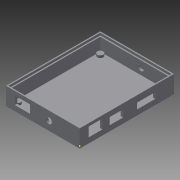
# Autodesk Inventor part: pcbProtectiveCase
Saved by Autodesk Inventor 2015 (Build 190159000, 159)
## iProperties
Created: 2015-02-12
Part Number: pcbProtectiveCase
Material: Generic
Document SubType Name: Modeling
Designer: 477grp12
Density: 1 g/cm^3
Appearance: Default
Author: 477grp12
Autodesk Inventor part; units mm, degrees
ref_plane "YZ Plane" through (0, 0, 0) normal (1, 0, 0) x (0, 1, 0)
ref_plane "XZ Plane" through (0, 0, 0) normal (0, 1, 0) x (-1, 0, 0)
ref_plane "XY Plane" through (0, 0, 0) normal (0, 0, 1) x (1, 0, 0)
sketch "Sketch1" plane through (0, 0, 0) normal (0, 1, 0) x (-1, 0, 0)
  line L0 (0, 0) -> (62.86, 0)
  line L1 (62.86, 0) -> (62.86, -80.39)
  line L2 (62.86, -80.39) -> (0, -80.39)
  line L3 (0, -80.39) -> (0, 0)
  line L4 (2, -2) -> (60.86, -2)
  line L5 (60.86, -2) -> (60.86, -78.39)
  line L6 (60.86, -78.39) -> (2, -78.39)
  line L7 (2, -78.39) -> (2, -2)
  dimension "d0" = 62.86
  dimension "d1" = 80.39
  dimension "d2" = 58.86
  dimension "d3" = 76.39
  dimension "d4" = 2
  dimension "d5" = 2
  constraints: 16 end point, 4 parallel, 2 horizontal, 2 perpendicular
  measures "d0" distance of L1.end L2.end
  measures "d1" distance of L2.end L0.start
  measures "d2" distance of L5.end L6.end
  measures "d3" distance of L4.end L5.end
  measures "d4" distance between parallel lines of L0 L4
  measures "d5" distance between parallel lines of L7 L3
extrude "Extrusion1" add sketch "Sketch1" along normal blind 15 contours L0 L1 L2 L3 | L4 L5 L6 L7
shell "Shell1" thickness 2 removed faces 1 at (-20.9533, 15, -26.7967)
sketch "Sketch2" plane through (-60.86, 2, -2) normal (0, 1, 0) x (1, 0, 0)
  point P0 (60.86, -2)
sketch "Sketch3" plane through (0, 15, 0) normal (0, 1, 0) x (1, 0, 0)
  line L0 (-60.86, 2) -> (-60.86, 78.39) projected
  line L1 (-60.86, 78.39) -> (-2, 78.39) projected
  line L2 (-2, 78.39) -> (-2, 2) projected
  line L3 (-2, 2) -> (-60.86, 2) projected
  line L4 (-62.86, 0) -> (0, 0) projected
  line L5 (0, 0) -> (0, 80.39) projected
  line L6 (0, 80.39) -> (-62.86, 80.39) projected
  line L7 (-62.86, 80.39) -> (-62.86, 0) projected
  line L8 (-61.86, 79.39) -> (-1, 79.39)
  line L9 (-1, 79.39) -> (-1, 1)
  line L10 (-1, 1) -> (-61.86, 1)
  line L11 (-61.86, 1) -> (-61.86, 79.39)
  dimension "d9" = 1
  dimension "d10" = 1
  dimension "d11" = 1
  dimension "d12" = 1
  constraints: 8 end point, 2 parallel, 1 horizontal, 1 perpendicular
  measures "d9" distance between parallel lines of L6 L8
  measures "d10" distance between parallel lines of L5 L9
  measures "d11" distance between parallel lines of L4 L10
  measures "d12" distance between parallel lines of L7 L11
extrude "Extrusion2" cut sketch "Sketch3" against normal blind 2 contours L8 L9 L10 L11
sketch "Sketch4" plane through (-60.86, 2, -2) normal (0, 1, 0) x (1, 0, 0)
  circle A0 centre (3, 73.39) radius 2.5
  circle A1 centre (55.86, 73.39) radius 2.5
  circle A2 centre (3, 3) radius 2.5
  circle A3 centre (55.86, 3) radius 2.5
  line L0 (60.86, 78.39) -> (-2, 78.39) projected
  line L1 (-2, 78.39) -> (-2, -2) projected
  line L2 (60.86, -2) -> (60.86, 78.39) projected
  line L3 (-2, -2) -> (60.86, -2) projected
  dimension "d15" = 5
  dimension "d16" = 5
  dimension "d17" = 5
  dimension "d18" = 5
  dimension "d19" = 5
  dimension "d20" = 5
  dimension "d21" = 5
  dimension "d22" = 5
  dimension "d23" = 5
  dimension "d24" = 5
  dimension "d25" = 5
  dimension "d26" = 5
  constraints: 4 centre point
  measures "d15" distance from line of L0 A0.centre
  measures "d16" distance from line of L1 A0.centre
  measures "d17" distance from line of L2 A1.centre
  measures "d18" distance from line of L0 A1.centre
  measures "d19" distance from line of L3 A3.centre
  measures "d20" distance from line of L2 A3.centre
  measures "d21" distance from line of L1 A2.centre
  measures "d22" distance from line of L3 A2.centre
  measures "d23" diameter of A0
  measures "d24" diameter of A2
  measures "d25" diameter of A3
  measures "d26" diameter of A1
extrude "Extrusion3" add sketch "Sketch4" along normal blind 2 contours A0 | A1 | A2 | A3
sketch "Sketch5" plane through (0, 0, 0) normal (1, 0, 0) x (0, 0, -1)
  line L0 (7.5, 4) -> (2.5, 4) projected
  line L1 (77.89, 4) -> (72.89, 4) projected
  line L2 (72.89, 2) -> (72.89, 4) projected
  line L3 (77.89, 2) -> (77.89, 4) projected
  line L4 (78.39, 2) -> (2, 2) projected
  line L5 (78.39, 2) -> (78.39, 13) projected
  line L6 (80.39, 0) -> (0, 0) projected
  line L7 (80.39, 0) -> (80.39, 15) projected
  line L8 (0, 15) -> (80.39, 15) projected
  line L9 (0, 0) -> (0, 15) projected
  line L10 (7.5, 2) -> (7.5, 4) projected
  line L11 (2, 2) -> (2, 13) projected
  line L12 (2.5, 2) -> (2.5, 4) projected
  line L13 (79.39, 13) -> (1, 13) projected
  line L14 (7.5, 12.508) -> (19.3903, 12.508)
  line L15 (19.3903, 12.508) -> (19.3903, 4.508)
  line L16 (19.3903, 4.508) -> (7.5, 4.508)
  line L17 (7.5, 4.508) -> (7.5, 12.508)
  line L18 (25.6078, 10.508) -> (36.9891, 10.508)
  line L19 (36.9891, 10.508) -> (36.9891, 4.508)
  line L20 (36.9891, 4.508) -> (25.6078, 4.508)
  line L21 (25.6078, 4.508) -> (25.6078, 10.508)
  line L22 (49.0027, 9.508) -> (64.4938, 9.508)
  line L23 (64.4938, 9.508) -> (64.4938, 4.508)
  line L24 (64.4938, 4.508) -> (49.0027, 4.508)
  line L25 (49.0027, 4.508) -> (49.0027, 9.508)
  dimension "d29" = 0.508
  dimension "d30" = 8
  dimension "d31" = 6
  dimension "d32" = 5
  constraints: 24 end point, 6 parallel, 3 horizontal, 3 perpendicular, 1 collinear, 1 point on line
  measures "d29" distance between parallel lines of L0 L16
  measures "d30" distance between parallel lines of L16 L14
  measures "d31" distance between parallel lines of L20 L18
  measures "d32" distance between parallel lines of L24 L22
extrude "Extrusion4" cut sketch "Sketch5" against normal blind 2 contours L14 L15 L16 L17 | L18 L19 L20 L21 | L22 L23 L24 L25
sketch "Sketch6" plane through (-62.86, 0, 0) normal (0, 0, 1) x (1, 0, 0)
  line L0 (60.86, 2) -> (2, 2) projected
  line L1 (7.5, 4) -> (2.5, 4) projected
  line L2 (7.5, 2) -> (7.5, 4) projected
  line L3 (2.5, 2) -> (2.5, 4) projected
  line L4 (60.86, 2) -> (60.86, 13) projected
  line L5 (60.36, 4) -> (55.36, 4) projected
  line L6 (55.36, 2) -> (55.36, 4) projected
  line L7 (60.36, 2) -> (60.36, 4) projected
  line L8 (2, 2) -> (2, 13) projected
  line L9 (61.86, 13) -> (1, 13) projected
  line L10 (7.5, 11.508) -> (20.3381, 11.508)
  line L11 (20.3381, 11.508) -> (20.3381, 4.508)
  line L12 (20.3381, 4.508) -> (7.5, 4.508)
  line L13 (7.5, 4.508) -> (7.5, 11.508)
  circle A0 centre (36.6004, 7.508) radius 2.5
  point P0 (62.86, 0)
  dimension "d35" = 0.508
  dimension "d36" = 7
  dimension "d37" = 5
  dimension "d38" = 5.508
  constraints: 8 end point, 2 parallel, 1 centre point, 1 horizontal, 1 perpendicular
  measures "d35" distance between parallel lines of L1 L12
  measures "d36" distance between parallel lines of L12 L10
  measures "d37" diameter of A0
  measures "d38" distance from line of L0 A0.centre
extrude "Extrusion5" cut sketch "Sketch6" against normal blind 2 contours L10 L11 L12 L13 | A0
sketch "Sketch7" plane through (0, 0, -80.39) normal (0, 0, -1) x (-1, 0, 0)
  circle A0 centre (26.2596, 7.508) radius 2.5 projected
  point P0 (0, 0)
extrude "Extrusion6" cut sketch "Sketch7" against normal blind 2
body "Solid1"
